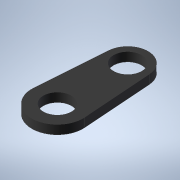
# Autodesk Inventor part: Piston
Saved by Autodesk Inventor 2022 (Build 260153000, 153)
## iProperties
Created: 2023-01-20
Part Number: Piston
Material: Generic
Document SubType Name: Modeling
Designer: ASUS
Density: 1 g/cm^3
Appearance: Default
Author: ASUS
Autodesk Inventor part; units mm, degrees
ref_plane "YZ Plane" through (0, 0, 0) normal (1, 0, 0) x (0, 1, 0)
ref_plane "XZ Plane" through (0, 0, 0) normal (0, 1, 0) x (-1, 0, 0)
ref_plane "XY Plane" through (0, 0, 0) normal (0, 0, 1) x (1, 0, 0)
sketch "Sketch1" plane through (0, 0, 0) normal (0, 1, 0) x (-1, 0, 0)
  arc A0 (19.9898, -0.6373) -> (-19.8657, -2.3139) centre (0, 0) ccw
  circle A1 centre (0, -55) radius 11.05
  line L0 (15, -86.1424) -> (-15, -86.1424) construction
  arc A2 (-15.9576, -56.1636) -> (15.9576, -56.1636) centre (0, -55) ccw
  circle A3 centre (0, 0) radius 11.05
  line L1 (21.1012, 14.3732) -> (11.6916, -114.6668)
  line L2 (-21.3969, 18.4288) -> (-13.9217, -84.0836)
  circle A4 centre (0, 0) radius 20
  point P0 (0, 0)
  point P1 (-19.947, -1.4545)
  point P2 (19.947, -1.4545)
  dimension "d1" = 40
  dimension "d2" = 22.1
  dimension "d6" = 0
  dimension "d7" = 32
  dimension "d8" = 22.1
  dimension "d12" = 55
  dimension "d13" = 0
  constraints: 6 end point, 4 centre point, 4 point on circle, 4 tangent, 3 coincident, 2 point on line, 1 horizontal, 3 other
  measures "d1" diameter of A0
  measures "d2" diameter of A1
  measures "d6" horizontal distance of A1.centre point (0, 0)
  measures "d7" diameter of A2
  measures "d8" diameter of A3
  measures "d12" distance of A1.centre point (0, 0)
  measures "d13" distance of point (0, 0) A0.centre
extrude "Extrusion1" add sketch "Sketch1" along normal blind 7
body "Solid1"
